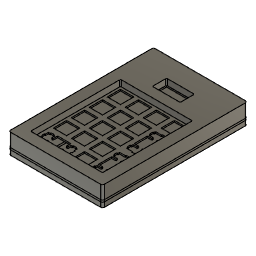
Numpadulator v15 (Autodesk Fusion 360 design; units mm, degrees)
Autodesk Fusion 360 part; units mm, degrees
(part 1 of 3)
sketch "998736cd7bd765a5d2f906dfe0ff0ee8913d12c1_switch" plane through (0, 0, 0) normal (0, 0, 1) x (1, 0, 0)
  line L0 (46.8697, 47.0546) -> (46.8697, 60.9053)
  line L1 (75.0701, 40.6054) -> (75.0701, 41.4295)
  line L2 (65.9197, 18.4795) -> (70.6191, 18.4795)
  line L3 (75.0701, 32.3301) -> (75.0701, 34.0045)
  line L4 (22.6191, 41.8553) -> (22.6191, 28.0045)
  line L5 (75.0701, 34.0045) -> (78.3001, 34.0045)
  line L6 (78.3001, 40.6054) -> (75.0701, 40.6054)
  line L7 (78.3001, 11.9297) -> (79.2194, 11.9297)
  line L8 (78.3001, 16.8052) -> (75.0701, 16.8052)
  line L9 (70.6191, 34.0045) -> (70.6191, 32.3301)
  line L10 (78.3001, 10.2044) -> (78.3001, 11.9297)
  line L11 (46.8697, 60.9053) -> (60.7191, 60.9053)
  line L12 (27.8198, 28.0045) -> (27.8198, 41.8553)
  line L13 (75.0701, 41.4295) -> (72.42, 41.4295)
  line L14 (60.7191, 41.8553) -> (60.7191, 28.0045)
  line L15 (70.6191, 18.4795) -> (70.6191, 16.8052)
  line L16 (70.6191, 32.3301) -> (65.9197, 32.3301)
  line L17 (8.7698, 28.0045) -> (8.7698, 41.8553)
  line L18 (27.8198, 41.8553) -> (41.6691, 41.8553)
  line L19 (65.1686, 15.0799) -> (65.1686, 11.9297)
  line L20 (65.1686, 11.9297) -> (66.1501, 11.9297)
  line L21 (78.3001, 35.7297) -> (79.2194, 35.7297)
  line L22 (79.2194, 38.88) -> (78.3001, 38.88)
  line L23 (66.1501, 11.9297) -> (66.1501, 10.2044)
  line L24 (79.2194, 15.0799) -> (78.3001, 15.0799)
  line L25 (78.3001, 38.88) -> (78.3001, 40.6054)
  line L26 (78.3001, 34.0045) -> (78.3001, 35.7297)
  line L27 (78.3001, 15.0799) -> (78.3001, 16.8052)
  line L28 (66.1501, 35.7297) -> (66.1501, 34.0045)
  line L29 (46.8697, 41.8553) -> (60.7191, 41.8553)
  line L30 (60.7191, 60.9053) -> (60.7191, 47.0546)
  line L31 (72.42, 10.2044) -> (72.42, 9.3803)
  line L32 (70.6191, 16.8052) -> (66.1501, 16.8052)
  line L33 (46.8697, 28.0045) -> (46.8697, 41.8553)
  line L34 (79.7691, 18.4795) -> (79.7691, 32.3301)
  line L35 (79.7691, 32.3301) -> (75.0701, 32.3301)
  line L36 (66.1501, 34.0045) -> (70.6191, 34.0045)
  line L37 (79.2194, 35.7297) -> (79.2194, 38.88)
  line L38 (66.1501, 15.0799) -> (65.1686, 15.0799)
  line L39 (17.2682, 122.266) -> (14.1194, 122.266)
  line L40 (14.1194, 109.197) -> (14.1194, 108.216)
  line L41 (37.3447, 108.967) -> (51.1941, 108.967)
  line L42 (51.1941, 108.967) -> (51.1941, 113.666)
  line L43 (14.1194, 108.216) -> (17.2682, 108.216)
  line L44 (8.7698, 99.0053) -> (22.6191, 99.0053)
  line L45 (37.3447, 122.816) -> (37.3447, 118.117)
  line L46 (17.2682, 121.347) -> (17.2682, 122.266)
  line L47 (69.5441, 121.347) -> (69.5441, 118.117)
  line L48 (11.57, 118.117) -> (11.57, 115.467)
  line L49 (71.2692, 108.216) -> (74.4181, 108.216)
  line L50 (69.5441, 109.197) -> (71.2692, 109.197)
  line L51 (76.145, 109.197) -> (76.145, 115.467)
  line L52 (76.9691, 118.117) -> (76.145, 118.117)
  line L53 (18.9949, 118.117) -> (18.9949, 121.347)
  line L54 (51.1941, 122.816) -> (37.3447, 122.816)
  line L55 (51.1941, 113.666) -> (69.5441, 113.666)
  line L56 (69.5441, 113.666) -> (69.5441, 109.197)
  line L57 (17.2682, 109.197) -> (18.9949, 109.197)
  line L58 (74.4181, 122.266) -> (71.2692, 122.266)
  line L59 (27.8198, 99.0053) -> (41.6691, 99.0053)
  line L60 (14.1194, 121.347) -> (12.3941, 121.347)
  line L61 (76.145, 115.467) -> (76.9691, 115.467)
  line L62 (71.2692, 121.347) -> (69.5441, 121.347)
  line L63 (37.3447, 118.117) -> (18.9949, 118.117)
  line L64 (76.145, 121.347) -> (74.4181, 121.347)
  line L65 (11.57, 115.467) -> (12.3941, 115.467)
  line L66 (14.1194, 122.266) -> (14.1194, 121.347)
  line L67 (17.2682, 108.216) -> (17.2682, 109.197)
  line L68 (76.145, 118.117) -> (76.145, 121.347)
  line L69 (71.2692, 109.197) -> (71.2692, 108.216)
  line L70 (41.6691, 99.0053) -> (41.6691, 85.1546)
  line L71 (18.9949, 113.666) -> (37.3447, 113.666)
  line L72 (12.3941, 115.467) -> (12.3941, 109.197)
  line L73 (71.2692, 122.266) -> (71.2692, 121.347)
  line L74 (74.4181, 109.197) -> (76.145, 109.197)
  line L75 (27.8198, 85.1546) -> (27.8198, 99.0053)
  line L76 (18.9949, 109.197) -> (18.9949, 113.666)
  line L77 (12.3941, 118.117) -> (11.57, 118.117)
  line L78 (12.3941, 121.347) -> (12.3941, 118.117)
  line L79 (74.4181, 121.347) -> (74.4181, 122.266)
  line L80 (22.6191, 85.1546) -> (8.7698, 85.1546)
  line L81 (8.7698, 85.1546) -> (8.7698, 99.0053)
  line L82 (37.3447, 113.666) -> (37.3447, 108.967)
  line L83 (12.3941, 109.197) -> (14.1194, 109.197)
  line L84 (41.6691, 85.1546) -> (27.8198, 85.1546)
  line L85 (69.5441, 118.117) -> (51.1941, 118.117)
  line L86 (18.9949, 121.347) -> (17.2682, 121.347)
  line L87 (51.1941, 118.117) -> (51.1941, 122.816)
  line L88 (74.4181, 108.216) -> (74.4181, 109.197)
  line L89 (22.6191, 99.0053) -> (22.6191, 85.1546)
  line L90 (76.9691, 115.467) -> (76.9691, 118.117)
  line L91 (65.1686, 73.8297) -> (66.1501, 73.8297)
  line L92 (65.9197, 85.1546) -> (65.9197, 99.0053)
  line L93 (27.8198, 79.9553) -> (41.6691, 79.9553)
  line L94 (41.6691, 79.9553) -> (41.6691, 66.1046)
  line L95 (75.0701, 54.9053) -> (75.0701, 56.5796)
  line L96 (75.0701, 56.5796) -> (79.7691, 56.5796)
  line L97 (75.0701, 78.7054) -> (75.0701, 79.5295)
  line L98 (79.2194, 73.8297) -> (79.2194, 76.98)
  line L99 (46.8697, 79.9553) -> (60.7191, 79.9553)
  line L100 (60.7191, 79.9553) -> (60.7191, 66.1046)
  line L101 (41.6691, 66.1046) -> (27.8198, 66.1046)
  line L102 (46.8697, 99.0053) -> (60.7191, 99.0053)
  line L103 (79.2194, 53.1798) -> (78.3001, 53.1798)
  line L104 (8.7698, 79.9553) -> (22.6191, 79.9553)
  line L105 (27.8198, 66.1046) -> (27.8198, 79.9553)
  line L106 (22.6191, 79.9553) -> (22.6191, 66.1046)
  line L107 (22.6191, 66.1046) -> (8.7698, 66.1046)
  line L108 (66.1501, 73.8297) -> (66.1501, 72.1046)
  line L109 (66.1501, 50.0295) -> (66.1501, 48.3044)
  line L110 (75.0701, 47.4804) -> (75.0701, 48.3044)
  line L111 (75.0701, 70.4303) -> (75.0701, 72.1046)
  line L112 (79.2194, 76.98) -> (78.3001, 76.98)
  line L113 (70.6191, 56.5796) -> (70.6191, 54.9053)
  line L114 (27.8198, 47.0546) -> (27.8198, 60.9053)
  line L115 (78.3001, 54.9053) -> (75.0701, 54.9053)
  line L116 (60.7191, 66.1046) -> (46.8697, 66.1046)
  line L117 (65.1686, 53.1798) -> (65.1686, 50.0295)
  line L118 (65.9197, 56.5796) -> (70.6191, 56.5796)
  line L119 (66.1501, 48.3044) -> (72.42, 48.3044)
  line L120 (65.9197, 99.0053) -> (79.7691, 99.0053)
  line L121 (66.1501, 53.1798) -> (65.1686, 53.1798)
  line L122 (22.6191, 60.9053) -> (22.6191, 47.0546)
  line L123 (70.6191, 72.1046) -> (70.6191, 70.4303)
  line L124 (79.7691, 99.0053) -> (79.7691, 85.1546)
  line L125 (72.42, 78.7054) -> (66.1501, 78.7054)
  line L126 (75.0701, 72.1046) -> (78.3001, 72.1046)
  line L127 (78.3001, 73.8297) -> (79.2194, 73.8297)
  line L128 (78.3001, 72.1046) -> (78.3001, 73.8297)
  line L129 (8.7698, 66.1046) -> (8.7698, 79.9553)
  line L130 (79.2194, 50.0295) -> (79.2194, 53.1798)
  line L131 (22.6191, 47.0546) -> (8.7698, 47.0546)
  line L132 (66.1501, 54.9053) -> (66.1501, 53.1798)
  line L133 (8.7698, 47.0546) -> (8.7698, 60.9053)
  line L134 (65.9197, 70.4303) -> (65.9197, 56.5796)
  line L135 (41.6691, 47.0546) -> (27.8198, 47.0546)
  line L136 (78.3001, 48.3044) -> (78.3001, 50.0295)
  line L137 (8.7698, 60.9053) -> (22.6191, 60.9053)
  line L138 (78.3001, 50.0295) -> (79.2194, 50.0295)
  line L139 (65.1686, 50.0295) -> (66.1501, 50.0295)
  line L140 (65.1686, 76.98) -> (65.1686, 73.8297)
  line L141 (78.3001, 53.1798) -> (78.3001, 54.9053)
  line L142 (66.1501, 76.98) -> (65.1686, 76.98)
  line L143 (72.42, 79.5295) -> (72.42, 78.7054)
  line L144 (72.42, 48.3044) -> (72.42, 47.4804)
  line L145 (79.7691, 70.4303) -> (75.0701, 70.4303)
  line L146 (79.7691, 56.5796) -> (79.7691, 70.4303)
  line L147 (46.8697, 66.1046) -> (46.8697, 79.9553)
  line L148 (75.0701, 79.5295) -> (72.42, 79.5295)
  line L149 (66.1501, 72.1046) -> (70.6191, 72.1046)
  line L150 (70.6191, 54.9053) -> (66.1501, 54.9053)
  line L151 (83.7691, 2.9545) -> (4.7713, 2.9545)
  line L152 (70.6191, 70.4303) -> (65.9197, 70.4303)
  line L153 (85.7691, 126.8149) -> (85.7691, 4.9545)
  line L154 (4.7713, 128.8149) -> (83.7691, 128.8149)
  line L155 (78.3001, 78.7054) -> (75.0701, 78.7054)
  line L156 (75.0701, 48.3044) -> (78.3001, 48.3044)
  line L157 (2.7713, 4.9545) -> (2.7713, 126.8149)
  line L158 (66.1501, 78.7054) -> (66.1501, 76.98)
  line L159 (72.42, 47.4804) -> (75.0701, 47.4804)
  line L160 (78.3001, 76.98) -> (78.3001, 78.7054)
  line L161 (18.2948, 22.8051) -> (18.2948, 18.1047)
  line L162 (11.745, 22.2539) -> (11.745, 21.3348)
  line L163 (10.0183, 18.1047) -> (9.1929, 18.1047)
  line L164 (9.1929, 15.4547) -> (10.0183, 15.4547)
  line L165 (11.745, 9.1846) -> (11.745, 8.2048)
  line L166 (14.8939, 9.1846) -> (16.6192, 9.1846)
  line L167 (14.8939, 8.2048) -> (14.8939, 9.1846)
  line L168 (9.1929, 18.1047) -> (9.1929, 15.4547)
  line L169 (16.6192, 21.3348) -> (14.8939, 21.3348)
  line L170 (11.745, 8.2048) -> (14.8939, 8.2048)
  line L171 (16.6192, 9.1846) -> (16.6192, 13.655)
  line L172 (14.8939, 22.2539) -> (11.745, 22.2539)
  line L173 (18.2948, 18.1047) -> (16.6192, 18.1047)
  line L174 (14.8939, 21.3348) -> (14.8939, 22.2539)
  line L175 (11.745, 21.3348) -> (10.0183, 21.3348)
  line L176 (16.6192, 18.1047) -> (16.6192, 21.3348)
  line L177 (10.0183, 21.3348) -> (10.0183, 18.1047)
  line L178 (10.0183, 15.4547) -> (10.0183, 9.1846)
  line L179 (10.0183, 9.1846) -> (11.745, 9.1846)
  line L180 (41.2447, 15.4547) -> (41.2447, 18.1047)
  line L181 (16.6192, 13.655) -> (18.2948, 13.655)
  line L182 (38.6941, 21.3348) -> (38.6941, 22.2539)
  line L183 (32.1441, 18.1047) -> (32.1441, 22.8051)
  line L184 (33.8198, 21.3348) -> (33.8198, 18.1047)
  line L185 (32.1441, 22.8051) -> (18.2948, 22.8051)
  line L186 (72.42, 41.4295) -> (72.42, 40.6054)
  line L187 (46.8697, 22.8051) -> (60.7191, 22.8051)
  line L188 (60.7191, 8.9545) -> (46.8697, 8.9545)
  line L189 (66.1501, 40.6054) -> (66.1501, 38.88)
  line L190 (66.1501, 38.88) -> (65.1686, 38.88)
  line L191 (40.4192, 9.1846) -> (40.4192, 15.4547)
  line L192 (33.8198, 13.655) -> (33.8198, 9.1846)
  line L193 (41.2447, 18.1047) -> (40.4192, 18.1047)
  line L194 (40.4192, 21.3348) -> (38.6941, 21.3348)
  line L195 (65.1686, 38.88) -> (65.1686, 35.7297)
  line L196 (18.2948, 8.9545) -> (32.1441, 8.9545)
  line L197 (38.6941, 22.2539) -> (35.5452, 22.2539)
  line L198 (72.42, 40.6054) -> (66.1501, 40.6054)
  line L199 (65.1686, 35.7297) -> (66.1501, 35.7297)
  line L200 (60.7191, 22.8051) -> (60.7191, 8.9545)
  line L201 (35.5452, 21.3348) -> (33.8198, 21.3348)
  line L202 (38.6941, 9.1846) -> (40.4192, 9.1846)
  line L203 (18.2948, 13.655) -> (18.2948, 8.9545)
  line L204 (33.8198, 9.1846) -> (35.5452, 9.1846)
  line L205 (32.1441, 8.9545) -> (32.1441, 13.655)
  line L206 (40.4192, 15.4547) -> (41.2447, 15.4547)
  line L207 (35.5452, 9.1846) -> (35.5452, 8.2048)
  line L208 (32.1441, 13.655) -> (33.8198, 13.655)
  line L209 (35.5452, 8.2048) -> (38.6941, 8.2048)
  line L210 (60.7191, 28.0045) -> (46.8697, 28.0045)
  line L211 (41.6691, 41.8553) -> (41.6691, 28.0045)
  line L212 (40.4192, 18.1047) -> (40.4192, 21.3348)
  line L213 (35.5452, 22.2539) -> (35.5452, 21.3348)
  line L214 (33.8198, 18.1047) -> (32.1441, 18.1047)
  line L215 (38.6941, 8.2048) -> (38.6941, 9.1846)
  line L216 (46.8697, 8.9545) -> (46.8697, 22.8051)
  line L217 (75.0701, 18.4795) -> (79.7691, 18.4795)
  line L218 (72.42, 9.3803) -> (75.0701, 9.3803)
  line L219 (8.7698, 41.8553) -> (22.6191, 41.8553)
  line L220 (41.6691, 28.0045) -> (27.8198, 28.0045)
  line L221 (60.7191, 47.0546) -> (46.8697, 47.0546)
  line L222 (75.0701, 9.3803) -> (75.0701, 10.2044)
  line L223 (22.6191, 28.0045) -> (8.7698, 28.0045)
  line L224 (27.8198, 60.9053) -> (41.6691, 60.9053)
  line L225 (65.9197, 32.3301) -> (65.9197, 18.4795)
  line L226 (79.2194, 11.9297) -> (79.2194, 15.0799)
  line L227 (75.0701, 16.8052) -> (75.0701, 18.4795)
  line L228 (75.0701, 10.2044) -> (78.3001, 10.2044)
  line L229 (41.6691, 60.9053) -> (41.6691, 47.0546)
  line L230 (66.1501, 16.8052) -> (66.1501, 15.0799)
  line L231 (66.1501, 10.2044) -> (72.42, 10.2044)
  line L232 (60.7191, 99.0053) -> (60.7191, 85.1546)
  line L233 (60.7191, 85.1546) -> (46.8697, 85.1546)
  line L234 (79.7691, 85.1546) -> (65.9197, 85.1546)
  line L235 (46.8697, 85.1546) -> (46.8697, 99.0053)
  arc A0 (85.7691, 126.8149) -> (83.7691, 128.8149) centre (83.7691, 126.8149) ccw
  arc A1 (83.7691, 2.9545) -> (85.7691, 4.9545) centre (83.7691, 4.9545) ccw
  arc A2 (2.7713, 4.9545) -> (4.7713, 2.9545) centre (4.7713, 4.9545) ccw
  arc A3 (4.7713, 128.8149) -> (2.7713, 126.8149) centre (4.7713, 126.8149) ccw
  line L236 (85.7691, 65.8847) -> (2.7713, 65.8847) construction
  line L237 (44.2702, 128.8149) -> (44.2702, 2.9545) construction
  dimension "d11" = 2
  dimension "d12" = 2
  dimension "d13" = 2
  dimension "d14" = 2
  dimension "d34" = 6
  dimension "d35" = 6
  constraint tangent L154 A0
  constraint tangent L153 A0
  constraint tangent L151 A1
  constraint tangent L153 A1
  constraint tangent L151 A2
  constraint tangent L157 A2
  constraint tangent L154 A3
  constraint tangent L157 A3
  constraint midpoint L153 L236.start
  constraint midpoint L157 L236.end
  constraint perpendicular L157 L236
  constraint midpoint L154 L237.start
  constraint midpoint L151 L237.end
  constraint perpendicular L151 L237
  measures "d11" radius of A0
  measures "d12" radius of A1
  measures "d13" radius of A2
  measures "d14" radius of A3
  measures "d34" distance of L151 L188
  measures "d35" distance of L146 L153
sketch "Sketch1" plane through (0, 0, 0) normal (0, 0, 1) x (1, 0, 0) in component "Plate"
sketch "eaeb931b339a04fc4a439f0e48c97f53086cf32d_switch" plane through (0, 0, 0) normal (0, 0, 1) x (1, 0, 0) in component "Plate"
  line L0 (20.1442, 10.8355) -> (34.145, 10.8355)
  line L1 (11.869, 23.3646) -> (11.869, 20.1345)
  line L2 (16.8934, 11.0657) -> (18.6201, 11.0657)
  line L3 (85.77, 4.8355) -> (6.6192, 4.8355)
  line L4 (40.6936, 10.0858) -> (40.6936, 11.0657)
  line L5 (13.593, 24.2852) -> (13.593, 23.3646)
  line L6 (37.3944, 10.0858) -> (40.6936, 10.0858)
  line L7 (42.4187, 17.3357) -> (43.2442, 17.3357)
  line L8 (20.1442, 20.1345) -> (18.6201, 20.1345)
  line L9 (42.4187, 11.0657) -> (42.4187, 17.3357)
  line L10 (16.8934, 23.3646) -> (16.8934, 24.2852)
  line L11 (37.3944, 11.0657) -> (37.3944, 10.0858)
  line L12 (11.0436, 20.1345) -> (11.0436, 17.3357)
  line L13 (40.6936, 11.0657) -> (42.4187, 11.0657)
  line L14 (6.6192, 142.035) -> (85.77, 142.035)
  line L15 (11.869, 17.3357) -> (11.869, 11.0657)
  line L16 (18.6201, 20.1345) -> (18.6201, 23.3646)
  line L17 (20.1442, 15.5346) -> (20.1442, 10.8355)
  line L18 (35.669, 11.0657) -> (37.3944, 11.0657)
  line L19 (74.2692, 42.635) -> (67.9993, 42.635)
  line L20 (67.9993, 42.635) -> (67.9993, 40.9099)
  line L21 (16.8934, 10.0858) -> (16.8934, 11.0657)
  line L22 (67.0197, 40.9099) -> (67.0197, 37.6107)
  line L23 (67.7693, 34.36) -> (67.7693, 20.3605)
  line L24 (74.2692, 81.5605) -> (74.2692, 80.735)
  line L25 (67.0197, 13.8107) -> (67.9993, 13.8107)
  line L26 (34.145, 24.835) -> (20.1442, 24.835)
  line L27 (48.7193, 10.8355) -> (48.7193, 24.835)
  line L28 (35.669, 20.1345) -> (34.145, 20.1345)
  line L29 (62.72, 10.8355) -> (48.7193, 10.8355)
  line L30 (67.9993, 37.6107) -> (67.9993, 35.8856)
  line L31 (18.6201, 11.0657) -> (18.6201, 15.5346)
  line L32 (67.7693, 20.3605) -> (72.4697, 20.3605)
  line L33 (43.2442, 17.3357) -> (43.2442, 20.1345)
  line L34 (18.6201, 15.5346) -> (20.1442, 15.5346)
  line L35 (77.0696, 11.26) -> (77.0696, 12.0854)
  line L36 (67.9993, 17.1097) -> (67.0197, 17.1097)
  line L37 (72.4697, 35.8856) -> (72.4697, 34.36)
  line L38 (67.0197, 17.1097) -> (67.0197, 13.8107)
  line L39 (29.6692, 29.8855) -> (29.6692, 43.8849)
  line L40 (10.6192, 43.8849) -> (24.62, 43.8849)
  line L41 (67.9993, 12.0854) -> (74.2692, 12.0854)
  line L42 (18.6201, 23.3646) -> (16.8934, 23.3646)
  line L43 (81.219, 40.9099) -> (80.2996, 40.9099)
  line L44 (62.72, 43.8849) -> (62.72, 29.8855)
  line L45 (35.669, 15.5346) -> (35.669, 11.0657)
  line L46 (43.67, 43.8849) -> (43.67, 29.8855)
  line L47 (11.869, 11.0657) -> (13.593, 11.0657)
  line L48 (80.2996, 40.9099) -> (80.2996, 42.635)
  line L49 (37.3944, 23.3646) -> (35.669, 23.3646)
  line L50 (74.2692, 43.4605) -> (74.2692, 42.635)
  line L51 (34.145, 20.1345) -> (34.145, 24.835)
  line L52 (67.0197, 37.6107) -> (67.9993, 37.6107)
  line L53 (80.2996, 17.1097) -> (80.2996, 18.835)
  line L54 (72.4697, 34.36) -> (67.7693, 34.36)
  line L55 (77.0696, 35.8856) -> (80.2996, 35.8856)
  line L56 (13.593, 10.0858) -> (16.8934, 10.0858)
  line L57 (43.67, 48.9356) -> (29.6692, 48.9356)
  line L58 (77.0696, 18.835) -> (77.0696, 20.3605)
  line L59 (80.2996, 12.0854) -> (80.2996, 13.8107)
  line L60 (48.7193, 43.8849) -> (62.72, 43.8849)
  line L61 (42.4187, 23.3646) -> (40.6936, 23.3646)
  line L62 (40.6936, 24.2852) -> (37.3944, 24.2852)
  line L63 (20.1442, 24.835) -> (20.1442, 20.1345)
  line L64 (77.0696, 34.36) -> (77.0696, 35.8856)
  line L65 (87.77, 140.035) -> (87.77, 6.8355)
  line L66 (34.145, 10.8355) -> (34.145, 15.5346)
  line L67 (13.593, 23.3646) -> (11.869, 23.3646)
  line L68 (35.669, 23.3646) -> (35.669, 20.1345)
  line L69 (62.72, 24.835) -> (62.72, 10.8355)
  line L70 (42.4187, 20.1345) -> (42.4187, 23.3646)
  line L71 (67.9993, 40.9099) -> (67.0197, 40.9099)
  line L72 (11.0436, 17.3357) -> (11.869, 17.3357)
  line L73 (67.9993, 35.8856) -> (72.4697, 35.8856)
  line L74 (43.2442, 20.1345) -> (42.4187, 20.1345)
  line L75 (16.8934, 24.2852) -> (13.593, 24.2852)
  line L76 (4.6192, 6.8355) -> (4.6192, 140.035)
  line L77 (11.869, 20.1345) -> (11.0436, 20.1345)
  line L78 (48.7193, 24.835) -> (62.72, 24.835)
  line L79 (13.593, 11.0657) -> (13.593, 10.0858)
  line L80 (34.145, 15.5346) -> (35.669, 15.5346)
  line L81 (40.6936, 23.3646) -> (40.6936, 24.2852)
  line L82 (37.3944, 24.2852) -> (37.3944, 23.3646)
  line L83 (48.7193, 29.8855) -> (48.7193, 43.8849)
  line L84 (24.62, 43.8849) -> (24.62, 29.8855)
  line L85 (81.77, 87.0356) -> (67.7693, 87.0356)
  line L86 (48.7193, 48.9356) -> (48.7193, 62.9348)
  line L87 (72.4697, 56.9352) -> (67.9993, 56.9352)
  line L88 (43.67, 87.0356) -> (29.6692, 87.0356)
  line L89 (24.62, 81.9848) -> (24.62, 67.9856)
  line L90 (67.7693, 58.4606) -> (72.4697, 58.4606)
  line L91 (43.67, 81.9848) -> (43.67, 67.9856)
  line L92 (43.67, 101.035) -> (43.67, 87.0356)
  line L93 (77.0696, 73.9856) -> (80.2996, 73.9856)
  line L94 (77.0696, 49.36) -> (77.0696, 50.1855)
  line L95 (29.6692, 67.9856) -> (29.6692, 81.9848)
  line L96 (81.219, 75.7107) -> (81.219, 79.0099)
  line L97 (81.219, 51.9105) -> (81.219, 55.2097)
  line L98 (74.2692, 11.26) -> (77.0696, 11.26)
  line L99 (10.6192, 29.8855) -> (10.6192, 43.8849)
  line L100 (81.77, 101.035) -> (81.77, 87.0356)
  line L101 (80.2996, 75.7107) -> (81.219, 75.7107)
  line L102 (29.6692, 48.9356) -> (29.6692, 62.9348)
  line L103 (10.6192, 62.9348) -> (24.62, 62.9348)
  line L104 (29.6692, 101.035) -> (43.67, 101.035)
  line L105 (72.4697, 18.835) -> (67.9993, 18.835)
  line L106 (62.72, 29.8855) -> (48.7193, 29.8855)
  line L107 (80.2996, 55.2097) -> (80.2996, 56.9352)
  line L108 (80.2996, 13.8107) -> (81.219, 13.8107)
  line L109 (67.9993, 79.0099) -> (67.0197, 79.0099)
  line L110 (77.0696, 42.635) -> (77.0696, 43.4605)
  line L111 (74.2692, 12.0854) -> (74.2692, 11.26)
  line L112 (81.77, 20.3605) -> (81.77, 34.36)
  line L113 (24.62, 62.9348) -> (24.62, 48.9356)
  line L114 (48.7193, 62.9348) -> (62.72, 62.9348)
  line L115 (67.0197, 79.0099) -> (67.0197, 75.7107)
  line L116 (48.7193, 87.0356) -> (48.7193, 101.035)
  line L117 (80.2996, 37.6107) -> (81.219, 37.6107)
  line L118 (10.6192, 48.9356) -> (10.6192, 62.9348)
  line L119 (62.72, 48.9356) -> (48.7193, 48.9356)
  line L120 (80.2996, 42.635) -> (77.0696, 42.635)
  line L121 (24.62, 48.9356) -> (10.6192, 48.9356)
  line L122 (43.67, 67.9856) -> (29.6692, 67.9856)
  line L123 (67.9993, 80.735) -> (67.9993, 79.0099)
  line L124 (67.0197, 55.2097) -> (67.0197, 51.9105)
  line L125 (29.6692, 87.0356) -> (29.6692, 101.035)
  line L126 (80.2996, 18.835) -> (77.0696, 18.835)
  line L127 (74.2692, 80.735) -> (67.9993, 80.735)
  line L128 (81.219, 37.6107) -> (81.219, 40.9099)
  line L129 (77.0696, 12.0854) -> (80.2996, 12.0854)
  line L130 (43.67, 62.9348) -> (43.67, 48.9356)
  line L131 (43.67, 29.8855) -> (29.6692, 29.8855)
  line L132 (80.2996, 35.8856) -> (80.2996, 37.6107)
  line L133 (67.9993, 18.835) -> (67.9993, 17.1097)
  line L134 (24.62, 29.8855) -> (10.6192, 29.8855)
  line L135 (62.72, 62.9348) -> (62.72, 48.9356)
  line L136 (77.0696, 20.3605) -> (81.77, 20.3605)
  line L137 (81.77, 34.36) -> (77.0696, 34.36)
  line L138 (72.4697, 20.3605) -> (72.4697, 18.835)
  line L139 (81.219, 17.1097) -> (80.2996, 17.1097)
  line L140 (77.0696, 43.4605) -> (74.2692, 43.4605)
  line L141 (29.6692, 43.8849) -> (43.67, 43.8849)
  line L142 (81.219, 13.8107) -> (81.219, 17.1097)
  line L143 (67.9993, 13.8107) -> (67.9993, 12.0854)
  line L144 (29.6692, 62.9348) -> (43.67, 62.9348)
  line L145 (81.219, 79.0099) -> (80.2996, 79.0099)
  line L146 (62.72, 87.0356) -> (48.7193, 87.0356)
  line L147 (74.2692, 49.36) -> (77.0696, 49.36)
  line L148 (29.6692, 81.9848) -> (43.67, 81.9848)
  line L149 (10.6192, 101.035) -> (24.62, 101.035)
  line L150 (72.4697, 73.9856) -> (72.4697, 72.4598)
  line L151 (80.2996, 80.735) -> (77.0696, 80.735)
  line L152 (48.7193, 81.9848) -> (62.72, 81.9848)
  line L153 (81.219, 55.2097) -> (80.2996, 55.2097)
  line L154 (72.4697, 72.4598) -> (67.7693, 72.4598)
  line L155 (62.72, 81.9848) -> (62.72, 67.9856)
  line L156 (67.0197, 51.9105) -> (67.9993, 51.9105)
  line L157 (77.0696, 72.4598) -> (77.0696, 73.9856)
  line L158 (67.7693, 101.035) -> (81.77, 101.035)
  line L159 (67.7693, 72.4598) -> (67.7693, 58.4606)
  line L160 (24.62, 67.9856) -> (10.6192, 67.9856)
  line L161 (77.0696, 56.9352) -> (77.0696, 58.4606)
  line L162 (77.0696, 80.735) -> (77.0696, 81.5605)
  line L163 (48.7193, 101.035) -> (62.72, 101.035)
  line L164 (80.2996, 73.9856) -> (80.2996, 75.7107)
  line L165 (72.4697, 58.4606) -> (72.4697, 56.9352)
  line L166 (67.9993, 51.9105) -> (67.9993, 50.1855)
  line L167 (67.9993, 73.9856) -> (72.4697, 73.9856)
  line L168 (80.2996, 79.0099) -> (80.2996, 80.735)
  line L169 (74.2692, 50.1855) -> (74.2692, 49.36)
  line L170 (62.72, 67.9856) -> (48.7193, 67.9856)
  line L171 (67.9993, 75.7107) -> (67.9993, 73.9856)
  line L172 (67.9993, 56.9352) -> (67.9993, 55.2097)
  line L173 (67.0197, 75.7107) -> (67.9993, 75.7107)
  line L174 (67.9993, 50.1855) -> (74.2692, 50.1855)
  line L175 (81.77, 72.4598) -> (77.0696, 72.4598)
  line L176 (80.2996, 51.9105) -> (81.219, 51.9105)
  line L177 (10.6192, 81.9848) -> (24.62, 81.9848)
  line L178 (67.9993, 55.2097) -> (67.0197, 55.2097)
  line L179 (48.7193, 67.9856) -> (48.7193, 81.9848)
  line L180 (77.0696, 50.1855) -> (80.2996, 50.1855)
  line L181 (80.2996, 50.1855) -> (80.2996, 51.9105)
  line L182 (67.7693, 87.0356) -> (67.7693, 101.035)
  line L183 (77.0696, 81.5605) -> (74.2692, 81.5605)
  line L184 (62.72, 101.035) -> (62.72, 87.0356)
  line L185 (77.0696, 58.4606) -> (81.77, 58.4606)
  line L186 (10.6192, 67.9856) -> (10.6192, 81.9848)
  line L187 (80.2996, 56.9352) -> (77.0696, 56.9352)
  line L188 (81.77, 58.4606) -> (81.77, 72.4598)
  line L189 (10.6192, 87.0356) -> (10.6192, 101.035)
  line L190 (24.62, 101.035) -> (24.62, 87.0356)
  line L191 (24.62, 87.0356) -> (10.6192, 87.0356)
  arc A0 (6.6192, 142.035) -> (4.6192, 140.035) centre (6.6192, 140.035) ccw
  arc A1 (87.77, 140.035) -> (85.77, 142.035) centre (85.77, 140.035) ccw
  arc A2 (85.77, 4.8355) -> (87.77, 6.8355) centre (85.77, 6.8355) ccw
  arc A3 (4.6192, 6.8355) -> (6.6192, 4.8355) centre (6.6192, 6.8355) ccw
  line L192 (31.4446, 129.035) -> (31.4446, 114.035)
  line L193 (31.4446, 114.035) -> (60.9446, 114.035)
  line L194 (60.9446, 114.035) -> (60.9446, 129.035)
  line L195 (60.9446, 129.035) -> (31.4446, 129.035)
  line L196 (10.6192, 114.5353) -> (24.62, 114.5353)
  line L197 (24.62, 114.5353) -> (24.62, 128.5347)
  line L198 (24.62, 128.5347) -> (10.6192, 128.5347)
  line L199 (10.6192, 128.5347) -> (10.6192, 114.5353)
  line L200 (67.7693, 114.5353) -> (81.77, 114.5353)
  line L201 (81.77, 114.5353) -> (81.77, 128.5347)
  line L202 (81.77, 128.5347) -> (67.7693, 128.5347)
  line L203 (67.7693, 128.5347) -> (67.7693, 114.5353)
  line L204 (46.1946, 142.035) -> (46.1946, 4.8355) construction
  line L205 (81.77, 121.535) -> (10.6192, 121.535) construction
  line L206 (87.77, 101.035) -> (4.6192, 101.035) construction
  line L207 (87.77, 121.535) -> (4.6192, 121.535) construction
  line L208 (28.1946, 138.035) -> (64.1946, 138.035)
  line L209 (64.1946, 138.035) -> (64.1946, 105.035)
  line L210 (64.1946, 105.035) -> (28.1946, 105.035)
  line L211 (28.1946, 105.035) -> (28.1946, 138.035)
  line L212 (4.6192, 103.56) -> (87.77, 103.56) construction
  dimension "d77" = 2
  dimension "d78" = 2
  dimension "d79" = 2
  dimension "d80" = 2
  dimension "d81" = 6
  dimension "d83" = 6
  dimension "d84" = 6
  dimension "d162" = 29.5
  dimension "d163" = 15
  dimension "d184" = 41
  dimension "d185" = 36
  dimension "d186" = 33
  dimension "d187" = 2.525
  constraint tangent L14 A0
  constraint tangent L76 A0
  constraint tangent L14 A1
  constraint tangent L65 A1
  constraint tangent L3 A2
  constraint tangent L65 A2
  constraint tangent L3 A3
  constraint tangent L76 A3
  constraint collinear L190 L197
  constraint collinear L189 L199
  constraint equal L190 L197
  constraint equal L149 L198
  constraint parallel L192 L194
  constraint parallel L193 L195
  constraint parallel L14 L195
  constraint collinear L100 L201
  constraint equal L182 L203
  constraint collinear L198 L202
  constraint equal L191 L196
  constraint equal L85 L200
  constraint midpoint L14 L204.start
  constraint midpoint L3 L204.end
  constraint symmetric L192 L194 L204
  constraint midpoint L201 L205.start
  constraint midpoint L199 L205.end
  constraint perpendicular L199 L205
  constraint symmetric L193 L195 L205
  constraint coincident L65 L206.start
  constraint coincident L76 L206.end
  constraint perpendicular L76 L206
  constraint coincident L65 L207.start
  constraint coincident L76 L207.end
  constraint perpendicular L76 L207
  constraint equal L158 L202
  constraint equal L100 L201
  constraint equal L189 L199
  constraint collinear L205 L207
  constraint perpendicular L209 L210
  constraint perpendicular L208 L211
  constraint perpendicular L208 L209
  constraint symmetric L207 L208 L210
  constraint symmetric L204 L209 L211
  constraint collinear L158 L206
  constraint coincident L76 L212.start
  constraint coincident L65 L212.end
  constraint perpendicular L65 L212
  measures "d77" radius of A0
  measures "d78" radius of A1
  measures "d79" radius of A2
  measures "d80" radius of A3
  measures "d81" distance of L3 L29
  measures "d83" distance of L65 L100
  measures "d84" distance of L76 L189
  measures "d162" distance of L192.end L193.end
  measures "d163" distance of L193.end L194.end
  measures "d184" distance of L14 L104
  measures "d185" distance of L208.start L208.end
  measures "d186" distance of L208.end L209.end
  measures "d187" distance of L158 L212
extrude "Extrude1" add sketch "eaeb931b339a04fc4a439f0e48c97f53086cf32d_switch" along normal blind 1.5 contours L3 L14 L65 L76 A0 A1 A2 A3 | L200 L201 L202 L203 | L208 L209 L210 L211 makes body 1 in component "Plate"
sketch "Sketch1 (2)" plane through (0, 4.8355, 0) normal (0, -1, 0) x (1, 0, 0) in component "Top"
  line L0 (6.6192, 0) -> (85.77, 0)
  line L1 (85.77, 0) -> (85.77, 1.5)
  line L2 (85.77, 1.5) -> (6.6192, 1.5)
  line L3 (6.6192, 1.5) -> (6.6192, 0)
  line L4 (46.1946, 0) -> (46.1946, 25.65) construction
  line L5 (87.92, -6) -> (95.92, -6)
  line L6 (95.92, -6) -> (95.92, 8.15)
  line L7 (95.92, 8.15) -> (-3.5308, 8.15)
  line L8 (-3.5308, 8.15) -> (-3.5308, -6)
  line L9 (-3.5308, -6) -> (4.4692, -6)
  line L10 (4.4692, -6) -> (4.4692, 1.65)
  line L11 (4.4692, 1.65) -> (87.92, 1.65)
  line L12 (87.92, -6) -> (87.92, 1.65)
  line L13 (87.77, 0) -> (87.77, 1.5) construction
  dimension "d88" = 0.15
  dimension "d89" = 0.15
  dimension "d90" = 6
  dimension "d91" = 6.5
  dimension "d92" = 8
  constraint midpoint L0 L4.start
  constraint perpendicular L2 L4
  constraint perpendicular L5 L6
  constraint perpendicular L6 L7
  constraint perpendicular L7 L8
  constraint perpendicular L6 L9
  constraint perpendicular L7 L10
  constraint perpendicular L6 L11
  constraint perpendicular L11 L12
  constraint symmetric L4 L6.end L7.end
  constraint symmetric L4 L5.end L8.end
  constraint symmetric L4 L5.start L9.end
  measures "d88" distance of L12 L13
  measures "d89" distance of L2 L11
  measures "d90" distance of L0 L5
  measures "d91" distance of L7 L11
  measures "d92" distance of L5.start L5.end
extrude "Extrude1'" add sketch "Sketch1 (2)" against normal up to surface (137.1995 mm away) separate body contours L5 L6 L7 L8 L9 L10 L11 L12 makes body 2 in component "Top"
move_face "OffsetFaces1" offset 0.15 1 faces at (60.1031, 4.8355, 5.9833) on bodies 2 in component "Top"
move_face "OffsetFaces2" offset 0.15 1 faces at (60.1031, 142.035, 5.9833) on bodies 2 in component "Top"
sketch "Sketch2" plane through (0, 4.6855, 0) normal (0, -1, 0) x (1, 0, 0) in component "Top"
  line L0 (95.92, -6) -> (95.92, 8.15)
  line L1 (95.92, 8.15) -> (-3.5308, 8.15)
  line L2 (-3.5308, 8.15) -> (-3.5308, -6)
  line L3 (-3.5308, -6) -> (4.4692, -6)
  line L4 (4.4692, -6) -> (4.4692, 1.65)
  line L5 (4.4692, 1.65) -> (87.92, 1.65)
  line L6 (87.92, 1.65) -> (87.92, -6)
  line L7 (87.92, -6) -> (95.92, -6)
  line L8 (4.4692, -6) -> (87.92, -6)
  constraint coincident L3.end L4.start
  constraint coincident L6.end L7.start
extrude "Extrude2" add sketch "Sketch2" along normal blind 8 bodies 2 in component "Top"
sketch "Sketch3" plane through (0, 142.185, 0) normal (0, 1, 0) x (-1, 0, 0) in component "Top"
  line L0 (3.5308, 8.15) -> (-95.92, 8.15)
  line L1 (-95.92, 8.15) -> (-95.92, -6)
  line L2 (-95.92, -6) -> (-87.92, -6)
  line L3 (-87.92, -6) -> (-87.92, 1.65)
  line L4 (-87.92, 1.65) -> (-4.4692, 1.65)
  line L5 (-4.4692, 1.65) -> (-4.4692, -6)
  line L6 (-4.4692, -6) -> (3.5308, -6)
  line L7 (3.5308, -6) -> (3.5308, 8.15)
  line L8 (-87.92, -6) -> (-4.4692, -6)
  constraint coincident L2.end L3.start
  constraint coincident L5.end L6.start
extrude "Extrude3" add sketch "Sketch3" along normal blind 8 bodies 2 in component "Top"
sketch "Sketch3 (2)" plane through (0, 0, 1.5) normal (0, 0, 1) x (-1, 0, 0) in component "Plate"
  line L0 (-29.6692, -48.9356) -> (-29.6692, -62.9348)
  line L1 (-29.6692, -62.9348) -> (-43.67, -62.9348)
  line L2 (-43.67, -62.9348) -> (-43.67, -48.9356)
  line L3 (-43.67, -48.9356) -> (-29.6692, -48.9356)
  line L4 (-29.6692, -67.9856) -> (-29.6692, -81.9848)
  line L5 (-29.6692, -81.9848) -> (-43.67, -81.9848)
  line L6 (-43.67, -81.9848) -> (-43.67, -67.9856)
  line L7 (-43.67, -67.9856) -> (-29.6692, -67.9856)
  line L8 (-62.72, -67.9856) -> (-48.7193, -67.9856)
  line L9 (-48.7193, -67.9856) -> (-48.7193, -81.9848)
  line L10 (-48.7193, -81.9848) -> (-62.72, -81.9848)
  line L11 (-62.72, -81.9848) -> (-62.72, -67.9856)
  line L12 (-81.77, -87.0356) -> (-67.7693, -87.0356)
  line L13 (-67.7693, -87.0356) -> (-67.7693, -101.035)
  line L14 (-67.7693, -101.035) -> (-81.77, -101.035)
  line L15 (-81.77, -101.035) -> (-81.77, -87.0356)
  line L16 (-67.9993, -12.0854) -> (-67.9993, -13.8107)
  line L17 (-67.9993, -13.8107) -> (-67.0197, -13.8107)
  line L18 (-67.0197, -13.8107) -> (-67.0197, -17.1097)
  line L19 (-67.0197, -17.1097) -> (-67.9993, -17.1097)
  line L20 (-67.9993, -17.1097) -> (-67.9993, -18.835)
  line L21 (-67.9993, -18.835) -> (-72.4697, -18.835)
  line L22 (-72.4697, -18.835) -> (-72.4697, -20.3605)
  line L23 (-72.4697, -20.3605) -> (-67.7693, -20.3605)
  line L24 (-67.7693, -20.3605) -> (-67.7693, -34.36)
  line L25 (-67.7693, -34.36) -> (-72.4697, -34.36)
  line L26 (-72.4697, -34.36) -> (-72.4697, -35.8856)
  line L27 (-72.4697, -35.8856) -> (-67.9993, -35.8856)
  line L28 (-67.9993, -35.8856) -> (-67.9993, -37.6107)
  line L29 (-67.9993, -37.6107) -> (-67.0197, -37.6107)
  line L30 (-67.0197, -37.6107) -> (-67.0197, -40.9099)
  line L31 (-67.0197, -40.9099) -> (-67.9993, -40.9099)
  line L32 (-67.9993, -40.9099) -> (-67.9993, -42.635)
  line L33 (-67.9993, -42.635) -> (-74.2692, -42.635)
  line L34 (-74.2692, -42.635) -> (-74.2692, -43.4605)
  line L35 (-74.2692, -43.4605) -> (-77.0696, -43.4605)
  line L36 (-77.0696, -43.4605) -> (-77.0696, -42.635)
  line L37 (-77.0696, -42.635) -> (-80.2996, -42.635)
  line L38 (-80.2996, -42.635) -> (-80.2996, -40.9099)
  line L39 (-80.2996, -40.9099) -> (-81.219, -40.9099)
  line L40 (-81.219, -40.9099) -> (-81.219, -37.6107)
  line L41 (-81.219, -37.6107) -> (-80.2996, -37.6107)
  line L42 (-80.2996, -37.6107) -> (-80.2996, -35.8856)
  line L43 (-80.2996, -35.8856) -> (-77.0696, -35.8856)
  line L44 (-77.0696, -35.8856) -> (-77.0696, -34.36)
  line L45 (-77.0696, -34.36) -> (-81.77, -34.36)
  line L46 (-81.77, -34.36) -> (-81.77, -20.3605)
  line L47 (-81.77, -20.3605) -> (-77.0696, -20.3605)
  line L48 (-77.0696, -20.3605) -> (-77.0696, -18.835)
  line L49 (-77.0696, -18.835) -> (-80.2996, -18.835)
  line L50 (-80.2996, -18.835) -> (-80.2996, -17.1097)
  line L51 (-80.2996, -17.1097) -> (-81.219, -17.1097)
  line L52 (-81.219, -17.1097) -> (-81.219, -13.8107)
  line L53 (-81.219, -13.8107) -> (-80.2996, -13.8107)
  line L54 (-80.2996, -13.8107) -> (-80.2996, -12.0854)
  line L55 (-80.2996, -12.0854) -> (-77.0696, -12.0854)
  line L56 (-77.0696, -12.0854) -> (-77.0696, -11.26)
  line L57 (-77.0696, -11.26) -> (-74.2692, -11.26)
  line L58 (-74.2692, -11.26) -> (-74.2692, -12.0854)
  line L59 (-74.2692, -12.0854) -> (-67.9993, -12.0854)
  line L60 (-29.6692, -29.8855) -> (-29.6692, -43.8849)
  line L61 (-29.6692, -43.8849) -> (-43.67, -43.8849)
  line L62 (-43.67, -43.8849) -> (-43.67, -29.8855)
  line L63 (-43.67, -29.8855) -> (-29.6692, -29.8855)
  line L64 (-48.7193, -62.9348) -> (-62.72, -62.9348)
  line L65 (-62.72, -62.9348) -> (-62.72, -48.9356)
  line L66 (-62.72, -48.9356) -> (-48.7193, -48.9356)
  line L67 (-48.7193, -48.9356) -> (-48.7193, -62.9348)
  line L68 (-24.62, -43.8849) -> (-24.62, -29.8855)
  line L69 (-24.62, -29.8855) -> (-10.6192, -29.8855)
  line L70 (-10.6192, -29.8855) -> (-10.6192, -43.8849)
  line L71 (-10.6192, -43.8849) -> (-24.62, -43.8849)
  line L72 (-48.7193, -10.8355) -> (-48.7193, -24.835)
  line L73 (-48.7193, -24.835) -> (-62.72, -24.835)
  line L74 (-62.72, -24.835) -> (-62.72, -10.8355)
  line L75 (-62.72, -10.8355) -> (-48.7193, -10.8355)
  line L76 (-37.3944, -23.3646) -> (-37.3944, -24.2852)
  line L77 (-37.3944, -24.2852) -> (-40.6936, -24.2852)
  line L78 (-40.6936, -24.2852) -> (-40.6936, -23.3646)
  line L79 (-40.6936, -23.3646) -> (-42.4187, -23.3646)
  line L80 (-42.4187, -23.3646) -> (-42.4187, -20.1345)
  line L81 (-42.4187, -20.1345) -> (-43.2442, -20.1345)
  line L82 (-43.2442, -20.1345) -> (-43.2442, -17.3357)
  line L83 (-43.2442, -17.3357) -> (-42.4187, -17.3357)
  line L84 (-42.4187, -17.3357) -> (-42.4187, -11.0657)
  line L85 (-42.4187, -11.0657) -> (-40.6936, -11.0657)
  line L86 (-40.6936, -11.0657) -> (-40.6936, -10.0858)
  line L87 (-40.6936, -10.0858) -> (-37.3944, -10.0858)
  line L88 (-37.3944, -10.0858) -> (-37.3944, -11.0657)
  line L89 (-37.3944, -11.0657) -> (-35.669, -11.0657)
  line L90 (-35.669, -11.0657) -> (-35.669, -15.5346)
  line L91 (-35.669, -15.5346) -> (-34.145, -15.5346)
  line L92 (-34.145, -15.5346) -> (-34.145, -10.8355)
  line L93 (-34.145, -10.8355) -> (-20.1442, -10.8355)
  line L94 (-20.1442, -10.8355) -> (-20.1442, -15.5346)
  line L95 (-20.1442, -15.5346) -> (-18.6201, -15.5346)
  line L96 (-18.6201, -15.5346) -> (-18.6201, -11.0657)
  line L97 (-18.6201, -11.0657) -> (-16.8934, -11.0657)
  line L98 (-16.8934, -11.0657) -> (-16.8934, -10.0858)
  line L99 (-16.8934, -10.0858) -> (-13.593, -10.0858)
  line L100 (-13.593, -10.0858) -> (-13.593, -11.0657)
  line L101 (-13.593, -11.0657) -> (-11.869, -11.0657)
  line L102 (-11.869, -11.0657) -> (-11.869, -17.3357)
  line L103 (-11.869, -17.3357) -> (-11.0436, -17.3357)
  line L104 (-11.0436, -17.3357) -> (-11.0436, -20.1345)
  line L105 (-11.0436, -20.1345) -> (-11.869, -20.1345)
  line L106 (-11.869, -20.1345) -> (-11.869, -23.3646)
  line L107 (-11.869, -23.3646) -> (-13.593, -23.3646)
  line L108 (-13.593, -23.3646) -> (-13.593, -24.2852)
  line L109 (-13.593, -24.2852) -> (-16.8934, -24.2852)
  line L110 (-16.8934, -24.2852) -> (-16.8934, -23.3646)
  line L111 (-16.8934, -23.3646) -> (-18.6201, -23.3646)
  line L112 (-18.6201, -23.3646) -> (-18.6201, -20.1345)
  line L113 (-18.6201, -20.1345) -> (-20.1442, -20.1345)
  line L114 (-20.1442, -20.1345) -> (-20.1442, -24.835)
  line L115 (-20.1442, -24.835) -> (-34.145, -24.835)
  line L116 (-34.145, -24.835) -> (-34.145, -20.1345)
  line L117 (-34.145, -20.1345) -> (-35.669, -20.1345)
  line L118 (-35.669, -20.1345) -> (-35.669, -23.3646)
  line L119 (-35.669, -23.3646) -> (-37.3944, -23.3646)
  line L120 (-62.72, -43.8849) -> (-62.72, -29.8855)
  line L121 (-62.72, -29.8855) -> (-48.7193, -29.8855)
  line L122 (-48.7193, -29.8855) -> (-48.7193, -43.8849)
  line L123 (-48.7193, -43.8849) -> (-62.72, -43.8849)
  line L124 (-43.67, -87.0356) -> (-29.6692, -87.0356)
  line L125 (-29.6692, -87.0356) -> (-29.6692, -101.035)
  line L126 (-29.6692, -101.035) -> (-43.67, -101.035)
  line L127 (-43.67, -101.035) -> (-43.67, -87.0356)
  line L128 (-24.62, -62.9348) -> (-24.62, -48.9356)
  line L129 (-24.62, -48.9356) -> (-10.6192, -48.9356)
  line L130 (-10.6192, -48.9356) -> (-10.6192, -62.9348)
  line L131 (-10.6192, -62.9348) -> (-24.62, -62.9348)
  line L132 (-48.7193, -101.035) -> (-62.72, -101.035)
  line L133 (-62.72, -101.035) -> (-62.72, -87.0356)
  line L134 (-62.72, -87.0356) -> (-48.7193, -87.0356)
  line L135 (-48.7193, -87.0356) -> (-48.7193, -101.035)
  line L136 (-31.4446, -129.035) -> (-60.9446, -129.035)
  line L137 (-60.9446, -129.035) -> (-60.9446, -114.035)
  line L138 (-60.9446, -114.035) -> (-31.4446, -114.035)
  line L139 (-31.4446, -114.035) -> (-31.4446, -129.035)
  line L140 (-24.62, -101.035) -> (-24.62, -87.0356)
  line L141 (-24.62, -87.0356) -> (-10.6192, -87.0356)
  line L142 (-10.6192, -87.0356) -> (-10.6192, -101.035)
  line L143 (-10.6192, -101.035) -> (-24.62, -101.035)
  line L144 (-81.77, -72.4598) -> (-81.77, -58.4606)
  line L145 (-81.77, -58.4606) -> (-77.0696, -58.4606)
  line L146 (-77.0696, -58.4606) -> (-77.0696, -56.9352)
  line L147 (-77.0696, -56.9352) -> (-80.2996, -56.9352)
  line L148 (-80.2996, -56.9352) -> (-80.2996, -55.2097)
  line L149 (-80.2996, -55.2097) -> (-81.219, -55.2097)
  line L150 (-81.219, -55.2097) -> (-81.219, -51.9105)
  line L151 (-81.219, -51.9105) -> (-80.2996, -51.9105)
  line L152 (-80.2996, -51.9105) -> (-80.2996, -50.1855)
  line L153 (-80.2996, -50.1855) -> (-77.0696, -50.1855)
  line L154 (-77.0696, -50.1855) -> (-77.0696, -49.36)
  line L155 (-77.0696, -49.36) -> (-74.2692, -49.36)
  line L156 (-74.2692, -49.36) -> (-74.2692, -50.1855)
  line L157 (-74.2692, -50.1855) -> (-67.9993, -50.1855)
  line L158 (-67.9993, -50.1855) -> (-67.9993, -51.9105)
  line L159 (-67.9993, -51.9105) -> (-67.0197, -51.9105)
  line L160 (-67.0197, -51.9105) -> (-67.0197, -55.2097)
  line L161 (-67.0197, -55.2097) -> (-67.9993, -55.2097)
  line L162 (-67.9993, -55.2097) -> (-67.9993, -56.9352)
  line L163 (-67.9993, -56.9352) -> (-72.4697, -56.9352)
  line L164 (-72.4697, -56.9352) -> (-72.4697, -58.4606)
  line L165 (-72.4697, -58.4606) -> (-67.7693, -58.4606)
  line L166 (-67.7693, -58.4606) -> (-67.7693, -72.4598)
  line L167 (-67.7693, -72.4598) -> (-72.4697, -72.4598)
  line L168 (-72.4697, -72.4598) -> (-72.4697, -73.9856)
  line L169 (-72.4697, -73.9856) -> (-67.9993, -73.9856)
  line L170 (-67.9993, -73.9856) -> (-67.9993, -75.7107)
  line L171 (-67.9993, -75.7107) -> (-67.0197, -75.7107)
  line L172 (-67.0197, -75.7107) -> (-67.0197, -79.0099)
  line L173 (-67.0197, -79.0099) -> (-67.9993, -79.0099)
  line L174 (-67.9993, -79.0099) -> (-67.9993, -80.735)
  line L175 (-67.9993, -80.735) -> (-74.2692, -80.735)
  line L176 (-74.2692, -80.735) -> (-74.2692, -81.5605)
  line L177 (-74.2692, -81.5605) -> (-77.0696, -81.5605)
  line L178 (-77.0696, -81.5605) -> (-77.0696, -80.735)
  line L179 (-77.0696, -80.735) -> (-80.2996, -80.735)
  line L180 (-80.2996, -80.735) -> (-80.2996, -79.0099)
  line L181 (-80.2996, -79.0099) -> (-81.219, -79.0099)
  line L182 (-81.219, -79.0099) -> (-81.219, -75.7107)
  line L183 (-81.219, -75.7107) -> (-80.2996, -75.7107)
  line L184 (-80.2996, -75.7107) -> (-80.2996, -73.9856)
  line L185 (-80.2996, -73.9856) -> (-77.0696, -73.9856)
  line L186 (-77.0696, -73.9856) -> (-77.0696, -72.4598)
  line L187 (-77.0696, -72.4598) -> (-81.77, -72.4598)
  line L188 (-24.62, -67.9856) -> (-10.6192, -67.9856)
  line L189 (-10.6192, -67.9856) -> (-10.6192, -81.9848)
  line L190 (-10.6192, -81.9848) -> (-24.62, -81.9848)
  line L191 (-24.62, -81.9848) -> (-24.62, -67.9856)
  arc A0 (-6.6192, -142.035) -> (-4.6192, -140.035) centre (-6.6192, -140.035) ccw
  line L192 (-4.6192, -140.035) -> (-4.6192, -6.8355)
  arc A1 (-4.6192, -6.8355) -> (-6.6192, -4.8355) centre (-6.6192, -6.8355) ccw
  line L193 (-6.6192, -4.8355) -> (-85.77, -4.8355)
  arc A2 (-85.77, -4.8355) -> (-87.77, -6.8355) centre (-85.77, -6.8355) ccw
  line L194 (-87.77, -6.8355) -> (-87.77, -140.035)
  arc A3 (-87.77, -140.035) -> (-85.77, -142.035) centre (-85.77, -140.035) ccw
  line L195 (-85.77, -142.035) -> (-6.6192, -142.035)
  line L196 (-9.0946, -103.5603) -> (-83.2947, -103.5603)
  line L197 (-84.2947, -102.5603) -> (-84.2947, -9.3102)
  line L198 (-83.2947, -8.3103) -> (-9.0946, -8.3102)
  line L199 (-8.0946, -9.3102) -> (-8.0946, -102.5603)
  line L200 (-48.7193, -17.8353) -> (-62.72, -17.8353) construction
  line L201 (-74.7696, -101.035) -> (-74.7696, -87.0356) construction
  line L202 (-67.7693, -94.0353) -> (-81.77, -94.0353) construction
  line L203 (-17.6196, -101.035) -> (-17.6196, -87.0356) construction
  arc A4 (-84.2947, -102.5603) -> (-83.2947, -103.5603) centre (-83.2947, -102.5603) ccw
  arc A5 (-9.0946, -103.5603) -> (-8.0946, -102.5603) centre (-9.0946, -102.5603) ccw
  arc A6 (-83.2947, -8.3103) -> (-84.2947, -9.3102) centre (-83.2947, -9.3102) ccw
  arc A7 (-8.0946, -9.3102) -> (-9.0946, -8.3102) centre (-9.0946, -9.3102) ccw
  line L204 (-10.6192, -114.5353) -> (-10.6192, -128.5347)
  line L205 (-10.6192, -128.5347) -> (-24.62, -128.5347)
  line L206 (-24.62, -128.5347) -> (-24.62, -114.5353)
  line L207 (-24.62, -114.5353) -> (-10.6192, -114.5353)
  dimension "d101" = 9.525
  dimension "d102" = 9.525
  dimension "d103" = 9.525
  dimension "d104" = 9.525
  dimension "d105" = 1
  dimension "d106" = 1
  dimension "d107" = 1
  dimension "d108" = 1
  constraint perpendicular L75 L197
  constraint perpendicular L70 L198
  constraint perpendicular L143 L199
  constraint midpoint L72 L200.start
  constraint midpoint L74 L200.end
  constraint midpoint L14 L201.start
  constraint midpoint L12 L201.end
  constraint midpoint L13 L202.start
  constraint midpoint L15 L202.end
  constraint midpoint L143 L203.start
  constraint midpoint L141 L203.end
  constraint tangent L196 A4
  constraint tangent L197 A4
  constraint tangent L196 A5
  constraint tangent L199 A5
  constraint tangent L197 A6
  constraint tangent L198 A6
  constraint tangent L198 A7
  constraint tangent L199 A7
  measures "d101" distance of L196 L202
  measures "d102" distance of L198 L200
  measures "d103" distance of L197 L201
  measures "d104" distance of L199 L203
  measures "d105" radius of A4
  measures "d106" radius of A5
  measures "d107" radius of A6
  measures "d108" radius of A7
extrude "Extrude4" cut sketch "Sketch3 (2)" along normal up to surface (6.65 mm away) contours L0 L1 L2 L3 | L4 L5 L6 L7 | L8 L9 L10 L11 | L12 L13 L14 L15 | L16 L17 L18 L19 L20 L21 L22 L23 L24 L25 L26 L27 L28 L29 L30 L31 L32 L33 L34 L35 L36 L37 L38 L39 L40 L41 L42 L43 L44 L45 L46 L47 L48 L49 L50 L51 L52 L53 L54 L55 L56 L57 L58 L59 | L60 L61 L62 L63 | L64 L65 L66 L67 | L68 L69 L70 L71 | L72 L73 L74 L75 | L76 L77 L78 L79 L80 L81 L82 L83 L84 L85 L86 L87 L88 L89 L90 L91 L92 L93 L94 L95 L96 L97 L98 L99 L100 L101 L102 L103 L104 L105 L106 L107 L108 L109 L110 L111 L112 L113 L114 L115 L116 L117 L118 L119 | L120 L121 L122 L123 | L124 L125 L126 L127 | L128 L129 L130 L131 | L132 L133 L134 L135 | L140 L141 L142 L143 | L144 L145 L146 L147 L148 L149 L150 L151 L152 L153 L154 L155 L156 L157 L158 L159 L160 L161 L162 L163 L164 L165 L166 L167 L168 L169 L170 L171 L172 L173 L174 L175 L176 L177 L178 L179 L180 L181 L182 L183 L184 L185 L186 L187 | L188 L189 L190 L191 | L196 L197 L198 L199 A4 A5 A6 A7 bodies 2 in component "Top"
fillet "Fillet1" radius 2 1 edges at (95.92, -3.3145, 1.075) on bodies 2 in component "Top"
fillet "Fillet2" radius 2 1 edges at (-3.5308, -3.3145, 1.075) on bodies 2 in component "Top"
fillet "Fillet3" radius 2 1 edges at (-3.5308, 150.185, 1.075) on bodies 2 in component "Top"
fillet "Fillet4" radius 2 1 edges at (95.92, 150.185, 1.075) on bodies 2 in component "Top"
sketch "Sketch1 (3)" plane through (0, 0, -6) normal (0, 0, -1) x (1, 0, 0) in component "Lit Stripe"
  arc A0 (93.92, -150.185) -> (95.92, -148.185) centre (93.92, -148.185) ccw
  line L0 (95.92, -148.185) -> (95.92, 1.3145)
  arc A1 (95.92, 1.3145) -> (93.92, 3.3145) centre (93.92, 1.3145) ccw
  line L1 (93.92, 3.3145) -> (-1.5308, 3.3145)
  arc A2 (-1.5308, 3.3145) -> (-3.5308, 1.3145) centre (-1.5308, 1.3145) ccw
  line L2 (-3.5308, 1.3145) -> (-3.5308, -148.185)
  arc A3 (-3.5308, -148.185) -> (-1.5308, -150.185) centre (-1.5308, -148.185) ccw
  line L3 (-1.5308, -150.185) -> (93.92, -150.185)
  line L4 (87.92, -142.185) -> (4.4692, -142.185)
  line L5 (4.4692, -142.185) -> (4.4692, -4.6855)
  line L6 (4.4692, -4.6855) -> (87.92, -4.6855)
  line L7 (87.92, -4.6855) -> (87.92, -142.185)
  line L8 (93.92, -150.185) -> (-1.5308, -150.185)
  arc A4 (-3.5308, -148.185) -> (-1.5308, -150.185) centre (-1.5308, -148.185) ccw
  line L9 (-3.5308, -148.185) -> (-3.5308, 1.3145)
  arc A5 (-1.5308, 3.3145) -> (-3.5308, 1.3145) centre (-1.5308, 1.3145) ccw
  line L10 (-1.5308, 3.3145) -> (93.92, 3.3145)
  arc A6 (95.92, 1.3145) -> (93.92, 3.3145) centre (93.92, 1.3145) ccw
  line L11 (95.92, 1.3145) -> (95.92, -148.185)
  arc A7 (93.92, -150.185) -> (95.92, -148.185) centre (93.92, -148.185) ccw
  line L12 (70.92, -125.185) -> (21.4692, -125.185)
  line L13 (70.92, -21.6855) -> (70.92, -125.185)
  line L14 (21.4692, -21.6855) -> (70.92, -21.6855)
  line L15 (21.4692, -125.185) -> (21.4692, -21.6855)
  dimension "d117" = 25
extrude "Extrude1''" add sketch "Sketch1 (3)" along normal blind 2 separate body contours A0 L0 A1 L1 A2 L2 A3 L3 L8 A4 L9 A5 L10 A6 L11 A7 | L4 L5 L6 L7 makes body 3 in component "Lit Stripe"
sketch "Sketch1 (4)" plane through (0, 0, -8) normal (0, 0, -1) x (1, 0, 0) in component "Bottom"
  line L0 (70.92, -125.185) -> (21.4692, -125.185)
  line L1 (21.4692, -125.185) -> (21.4692, -21.6855)
  line L2 (21.4692, -21.6855) -> (70.92, -21.6855)
  line L3 (70.92, -21.6855) -> (70.92, -125.185)
  arc A0 (-3.5308, -148.185) -> (-1.5308, -150.185) centre (-1.5308, -148.185) ccw
  line L4 (-1.5308, -150.185) -> (93.92, -150.185)
  arc A1 (93.92, -150.185) -> (95.92, -148.185) centre (93.92, -148.185) ccw
  line L5 (95.92, -148.185) -> (95.92, 1.3145)
  arc A2 (95.92, 1.3145) -> (93.92, 3.3145) centre (93.92, 1.3145) ccw
  line L6 (93.92, 3.3145) -> (-1.5308, 3.3145)
  arc A3 (-1.5308, 3.3145) -> (-3.5308, 1.3145) centre (-1.5308, 1.3145) ccw
  line L7 (-3.5308, 1.3145) -> (-3.5308, -148.185)
  line L8 (93.92, 3.3145) -> (-1.5308, 3.3145)
  line L9 (-3.5308, 1.3145) -> (-3.5308, -148.185)
  line L10 (-1.5308, -150.185) -> (93.92, -150.185)
  line L11 (95.92, -148.185) -> (95.92, 1.3145)
  arc A4 (-3.5308, -148.185) -> (-1.5308, -150.185) centre (-1.5308, -148.185) ccw
  arc A5 (93.92, -150.185) -> (95.92, -148.185) centre (93.92, -148.185) ccw
  arc A6 (95.92, 1.3145) -> (93.92, 3.3145) centre (93.92, 1.3145) ccw
  arc A7 (-1.5308, 3.3145) -> (-3.5308, 1.3145) centre (-1.5308, 1.3145) ccw
extrude "Extrude1'''" add sketch "Sketch1 (4)" along normal blind 5 separate body contours L0 L1 L2 L3 | A0 L4 A1 L5 A2 L6 A3 L7 L8 L9 L10 L11 A4 A5 A6 A7 makes body 4 in component "Bottom"